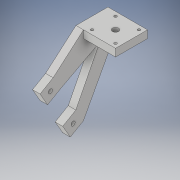
# Autodesk Inventor part: Stepper_Face
Saved by Autodesk Inventor 2019 (Build 230136000, 136)
## iProperties
Created: 2019-07-06
Part Number: Stepper_Face
Material: Generic
Document SubType Name: Modeling
Designer: Jorian Brusind
Density: 1 g/cm^3
Appearance: Default
Author: Jorian Brusind
Autodesk Inventor part; units mm, degrees
ref_plane "YZ Plane" through (0, 0, 0) normal (1, 0, 0) x (0, 1, 0)
ref_plane "XZ Plane" through (0, 0, 0) normal (0, 1, 0) x (-1, 0, 0)
ref_plane "XY Plane" through (0, 0, 0) normal (0, 0, 1) x (1, 0, 0)
sketch "Sketch1" plane through (0, 0, 0) normal (0, 1, 0) x (-1, 0, 0)
  line L0 (0, 0) -> (52.3, 0)
  line L1 (52.3, 0) -> (52.3, -42.3)
  line L2 (52.3, -42.3) -> (0, -42.3)
  line L3 (0, -42.3) -> (0, 0)
  dimension "d0" = 52.3
  dimension "d1" = 42.3
  constraints: 8 end point, 2 parallel, 1 horizontal, 1 perpendicular
  measures "d0" distance of L1.end L2.end
  measures "d1" distance of L0.end L1.end
extrude "Extrusion1" add sketch "Sketch1" along normal blind 10
sketch "Sketch2" plane through (0, 0, 0) normal (0, -1, 0) x (1, 0, 0)
  line L0 (-52.3, 0) -> (0, 0) projected
  line L1 (-52.3, 0) -> (-42.3, 0)
  line L2 (-42.3, 0) -> (-42.3, -42.3)
  line L3 (-42.3, -42.3) -> (-52.3, -42.3)
  line L4 (-52.3, -42.3) -> (-52.3, 0)
  dimension "d4" = 10
  dimension "d5" = 42.3
  constraints: 8 end point, 2 parallel, 1 horizontal, 1 perpendicular
  measures "d4" distance of L2.end L3.end
  measures "d5" distance of L1.end L2.end
extrude "Extrusion2" add sketch "Sketch2" along normal blind 15
sketch "Sketch3" plane through (0, 10, 0) normal (0, 1, 0) x (1, 0, 0)
  line L0 (0, 0) -> (0, 5.65)
  line L1 (0, 0) -> (0, 42.3) projected
  line L2 (0, 5.65) -> (-5.65, 5.65)
  circle A0 centre (-5.65, 5.65) radius 1.75
  circle A1 centre (-5.65, 36.65) radius 1.75
  circle A2 centre (-36.65, 5.65) radius 1.75
  circle A3 centre (-36.65, 36.65) radius 1.75
  dimension "d8" = 5.65
  dimension "d9" = 5.65
  dimension "d10" = 3.5
  dimension "d13" = 31
  dimension "d16" = 31
  constraints: 4 centre point, 4 end point, 1 coincident, 1 horizontal, 1 perpendicular, 1 point on line, 1 vertical, 6 other
  measures "d8" distance of L0.start L0.end
  measures "d9" distance of L0.end L2.end
  measures "d10" diameter of A0
  measures "d13" distance of A0.centre A1.centre
  measures "d16" distance of A0.centre A2.centre
extrude "Extrusion3" cut sketch "Sketch3" against normal blind 10
sketch "Sketch4" plane through (0, 10, 0) normal (0, 1, 0) x (1, 0, 0)
  line L0 (0, 42.3) -> (0, 0) projected
  line L1 (0, 21.15) -> (-21.15, 21.15)
  circle A0 centre (-21.15, 21.15) radius 4
  dimension "d21" = 21.15
  dimension "d22" = 8
  constraints: 2 end point, 1 centre point, 1 coincident, 1 horizontal, 1 midpoint
  measures "d21" distance of L1.start L1.end
  measures "d22" diameter of A0
extrude "Extrusion4" cut sketch "Sketch4" against normal blind 10
sketch "Sketch9" plane through (-52.3, 10, -42.3) normal (-1, 0, 0) x (0, 0, 1)
  line L0 (42.3, 0) -> (0, 0) projected
  line L1 (21.15, 0) -> (121.15, 0) construction
  line L2 (42.3, 0) -> (42.3, -25) projected
  line L3 (0, -25) -> (42.3, -25) projected
  line L4 (21.15, 0) -> (21.15, 12.2)
  line L5 (21.15, 12.2) -> (71.15, -74.4025)
  line L6 (21.15, 12.2) -> (121.15, 12.2) construction
  line L7 (71.15, -74.4025) -> (62.4897, -79.4025)
  line L8 (57.4897, -78.0628) -> (67.4897, -60.7423)
  line L9 (67.4897, -60.7423) -> (84.8103, -70.7423)
  line L10 (84.8103, -70.7423) -> (74.8103, -88.0628)
  line L11 (74.8103, -88.0628) -> (57.4897, -78.0628)
  line L12 (57.4897, -78.0628) -> (84.8103, -70.7423) construction
  line L13 (67.4897, -60.7423) -> (74.8103, -88.0628) construction
  line L14 (57.4897, -78.0628) -> (77.4897, -78.0628) construction
  line L15 (71.15, -74.4025) -> (86.15, -48.4218)
  line L16 (71.15, -74.4025) -> (101.15, -74.4025) construction
  circle A0 centre (86.15, -48.4218) radius 2.75
  line L17 (72.4897, -52.082) -> (82.4897, -34.7615)
  line L18 (82.4897, -34.7615) -> (99.8103, -44.7615)
  line L19 (99.8103, -44.7615) -> (89.8103, -62.082)
  line L20 (89.8103, -62.082) -> (72.4897, -52.082)
  line L21 (72.4897, -52.082) -> (99.8103, -44.7615) construction
  line L22 (82.4897, -34.7615) -> (89.8103, -62.082) construction
  line L23 (72.4897, -52.082) -> (92.4897, -52.082) construction
  line L24 (0, -10) -> (0, 0) projected
  line L25 (42.3, -25) -> (0, -25) projected
  line L26 (42.3, -10) -> (42.3, 0) projected
  line L27 (72.4897, -52.082) -> (21.15, -25)
  line L28 (42.3, -10) -> (42.3, -25) projected
  line L29 (0, -10) -> (0, -25) projected
  line L30 (42.4897, -104.0436) -> (52.4897, -86.723)
  line L31 (52.4897, -86.723) -> (69.8103, -96.723)
  line L32 (69.8103, -96.723) -> (59.8103, -114.0436)
  line L33 (59.8103, -114.0436) -> (42.4897, -104.0436)
  line L34 (42.4897, -104.0436) -> (69.8103, -96.723) construction
  circle A1 centre (56.15, -100.3833) radius 2.75
  line L35 (42.4897, -104.0436) -> (0, -25)
  line L36 (52.4897, -86.723) -> (21.15, -25)
  line L37 (72.4897, -52.082) -> (21.15, -25)
  line L38 (0, 0) -> (42.3, 0) projected
  line L39 (82.4897, -34.7615) -> (42.3, 0)
  dimension "d77" = 12.2
  dimension "d78" = 100
  dimension "d79" = 60
  dimension "d80" = 10
  dimension "d81" = 90
  dimension "d82" = 20
  dimension "d83" = 60
  dimension "d84" = 20
  dimension "d85" = 30
  dimension "d88" = 5.5
  dimension "d90" = 20
  dimension "d91" = 60
  dimension "d92" = 20
  dimension "d105" = 60
  constraints: 62 end point, 7 midpoint, 5 horizontal, 5 parallel, 3 equal length, 3 perpendicular, 2 centre point, 1 coincident, 1 collinear, 1 vertical, 12 other
  measures "d77" distance of L1.start L4.end
  measures "d78" distance of L4.end L5.end
  measures "d79" angle of L5 L6
  measures "d80" distance of L5.end L7.end
  measures "d81" angle of L5 L7
  measures "d82" distance of L8.start L8.end
  measures "d83" angle of L14 L8
  measures "d84" distance of L8.end L9.end
  measures "d85" distance of L5.end L15.end
  measures "d88" diameter of A0
  measures "d90" distance of L17.start L17.end
  measures "d91" angle of L23 L17
  measures "d92" distance of L17.end L18.end
  measures "d105" distance of L17.start L30.start
extrude "Extrusion10" add sketch "Sketch9" against normal blind 10 contours L39 L17 L27 L5 L2 | L5 L27 L3 L2 | L3 L36 L30 L35 | L18 L19 L20 L17 | L30 L31 L32 L33
body "Solid1"
